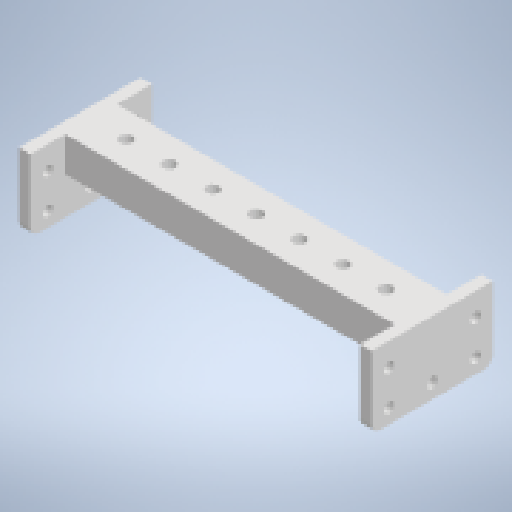
# Autodesk Inventor part: 加强梁
Saved by Autodesk Inventor 2025.1 (Build 291241000, 241)
## iProperties
Created: 2025-08-27
Part Number: 加强梁
Material: 常规
Document SubType Name: Modeling
Designer: Piw
Density: 1 g/cm^3
Appearance: 默认
Author: Piw
Autodesk Inventor part; units mm, degrees
ref_plane "YZ Plane" through (0, 0, 0) normal (1, 0, 0) x (0, 1, 0)
ref_plane "XZ Plane" through (0, 0, 0) normal (0, 1, 0) x (-1, 0, 0)
ref_plane "XY Plane" through (0, 0, 0) normal (0, 0, 1) x (1, 0, 0)
sketch "草图1" plane through (0, 0, 0) normal (1, 0, 0) x (0, 1, 0)
  line L0 (-12.5, 21) -> (12.5, 21)
  line L1 (12.5, 21) -> (12.5, -21)
  line L2 (12.5, -21) -> (-12.5, -21)
  line L3 (-12.5, -21) -> (-12.5, 21)
  line L4 (-12.5, 21) -> (12.5, -21) construction
  line L5 (12.5, 21) -> (-12.5, -21) construction
  line L6 (-7.5, -15) -> (4.5, -15) construction
  line L7 (4.5, -15) -> (4.5, 15) construction
  line L8 (4.5, 15) -> (-7.5, 15) construction
  line L9 (-7.5, 15) -> (-7.5, -15) construction
  line L10 (-7.5, -15) -> (4.5, 15) construction
  line L11 (4.5, -15) -> (-7.5, 15) construction
  line L12 (18.2853, 0) -> (0, 0) construction
  circle A0 centre (4.5, -15) radius 1.75
  circle A1 centre (4.5, 15) radius 1.75
  circle A2 centre (-7.5, 15) radius 1.75
  circle A3 centre (-7.5, 0) radius 1.75
  circle A4 centre (-7.5, -15) radius 1.75
  point P0 (-1.5, 0)
  dimension "d0" = 42
  dimension "d1" = 25
  dimension "d4" = 8
  dimension "d5" = 20
  dimension "d6" = 30
  dimension "d7" = 3.5
  dimension "d8" = 3.5
  dimension "d9" = 3.5
  dimension "d10" = 3.5
  dimension "d11" = 3.5
  constraints: 26 end point, 5 centre point, 5 midpoint, 4 coincident, 4 parallel, 3 horizontal, 2 perpendicular, 1 point on line
  measures "d0" distance of L2.end L0.start
  measures "d1" distance of L1.end L2.end
  measures "d4" distance between parallel lines of L1 L7
  measures "d5" distance between parallel lines of L9 L1
  measures "d6" distance of L8.end L6.start
  measures "d7" diameter of A0
  measures "d8" diameter of A1
  measures "d9" diameter of A2
  measures "d10" diameter of A3
  measures "d11" diameter of A4
extrude "拉伸1" add sketch "草图1" along normal blind 4
fillet "圆角1" radius 3 2 edges at (2, -12.5, -21) (2, -12.5, 21)
sketch "草图2" plane through (4, 0, 0) normal (1, 0, 0) x (0, 0, -1)
  line L0 (21, 12.5) -> (-21, 12.5) projected
  line L1 (9, -1.5) -> (-9, -1.5)
  line L2 (-9, -1.5) -> (-9, 12.5)
  line L3 (-9, 12.5) -> (9, 12.5)
  line L4 (9, 12.5) -> (9, -1.5)
  line L5 (9, -1.5) -> (-9, 12.5) construction
  line L6 (-9, -1.5) -> (9, 12.5) construction
  line L7 (0, -21.7484) -> (0, 21.3342) construction
  point P0 (0, 0)
  point P1 (0, 5.5)
  point P2 (9, 12.5)
  dimension "d15" = 18
  dimension "d16" = 14
  constraints: 14 end point, 2 midpoint, 2 parallel, 2 point on line, 2 vertical, 1 horizontal, 1 perpendicular
  measures "d15" distance between parallel lines of L4 L2
  measures "d16" distance between parallel lines of L0 L1
extrude "拉伸2" add sketch "草图2" along normal blind 114
sketch "草图3" plane through (118, 0, 0) normal (1, 0, 0) x (0, 0, -1)
  arc A0 (-21, -9.5) -> (-18, -12.5) centre (-18, -9.5) ccw projected
  line L0 (-21, 12.5) -> (-21, -9.5) projected
  line L1 (21, 12.5) -> (-21, 12.5) projected
  line L2 (21, -9.5) -> (21, 12.5) projected
  arc A1 (18, -12.5) -> (21, -9.5) centre (18, -9.5) ccw projected
  line L3 (-18, -12.5) -> (18, -12.5) projected
  circle A2 centre (15, -7.5) radius 1.75 projected
  circle A3 centre (0, -7.5) radius 1.75 projected
  circle A4 centre (-15, -7.5) radius 1.75 projected
  circle A5 centre (-15, 4.5) radius 1.75 projected
  circle A6 centre (15, 4.5) radius 1.75 projected
  point P0 (0, 0)
extrude "拉伸3" add sketch "草图3" along normal blind 4
chamfer "倒角1" distance 2 angle 45 2 edges at (61, -1.5, -9) (61, -1.5, 9)
sketch "草图4" plane through (0, 12.5, 21) normal (0, 1, 0) x (1, 0, 0)
  line L0 (61, 0.1174) -> (61, 41.8826) construction
  line L1 (122, 42) -> (122, 0) projected
  line L2 (0, 42) -> (0, 0) projected
  circle A0 centre (61, 21) radius 2.1
  line L3 (122, 21) -> (0, 21) construction
  circle A1 centre (46, 21) radius 2.1
  circle A2 centre (31, 21) radius 2.1
  circle A3 centre (16, 21) radius 2.1
  circle A4 centre (76, 21) radius 2.1
  circle A5 centre (61, 21) radius 2.1
  circle A6 centre (46, 21) radius 2.1
  circle A7 centre (31, 21) radius 2.1
  circle A8 centre (91, 21) radius 2.1
  circle A9 centre (76, 21) radius 2.1
  circle A10 centre (61, 21) radius 2.1
  circle A11 centre (46, 21) radius 2.1
  circle A12 centre (106, 21) radius 2.1
  circle A13 centre (91, 21) radius 2.1
  circle A14 centre (76, 21) radius 2.1
  circle A15 centre (61, 21) radius 2.1
  dimension "d24" = 61
  dimension "d25" = 61
  dimension "d26" = 4.2
  dimension "d29" = 15
  dimension "d32" = 15
  constraints: 16 centre point, 4 end point, 3 midpoint, 2 horizontal, 1 perpendicular, 1 vertical, 30 other
  measures "d24" distance between parallel lines of L1 L0
  measures "d25" distance between parallel lines of L2 L0
  measures "d26" diameter of A0
  measures "d29" distance of A0.centre A1.centre
  measures "d32" distance of A0.centre A4.centre
extrude "拉伸4" cut sketch "草图4" against normal through all
